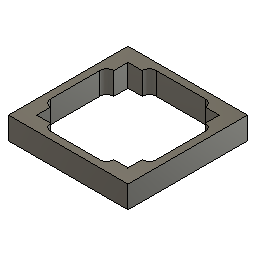
TinyNES_Foam_Bottom (Autodesk Fusion 360 design; units mm, degrees)
Autodesk Fusion 360 part; units mm, degrees
sketch "Sketch1" plane through (0, 0, 0) normal (0, 1, 0) x (1, 0, 0)
  line L0 (0, 0) -> (170, 0)
  line L1 (170, 0) -> (170, 170)
  line L2 (170, 170) -> (0, 170)
  line L3 (0, 170) -> (0, 0)
  line L4 (85, 0) -> (85, 170) construction
  line L5 (150, 150) -> (20, 150)
  line L6 (20, 150) -> (20, 20)
  line L7 (20, 20) -> (150, 20)
  line L8 (150, 20) -> (150, 150)
  line L9 (150, 150) -> (20, 20) construction
  line L10 (20, 150) -> (150, 20) construction
  line L11 (120, 160) -> (50, 160)
  line L12 (40, 150) -> (40, 20) construction
  line L13 (50, 10) -> (120, 10)
  line L14 (130, 20) -> (130, 150) construction
  line L15 (130, 160) -> (40, 10) construction
  line L16 (40, 160) -> (130, 10) construction
  line L17 (150, 130) -> (20, 130) construction
  line L18 (10, 120) -> (10, 50)
  line L19 (20, 40) -> (150, 40) construction
  line L20 (160, 50) -> (160, 120)
  line L21 (160, 130) -> (10, 40) construction
  line L22 (10, 130) -> (160, 40) construction
  arc A0 (50, 160) -> (40, 150) centre (50, 150) ccw
  arc A1 (130, 150) -> (120, 160) centre (120, 150) ccw
  arc A2 (160, 120) -> (150, 130) centre (150, 120) ccw
  arc A3 (150, 40) -> (160, 50) centre (150, 50) ccw
  arc A4 (120, 10) -> (130, 20) centre (120, 20) ccw
  arc A5 (40, 20) -> (50, 10) centre (50, 20) ccw
  arc A6 (10, 50) -> (20, 40) centre (20, 50) ccw
  arc A7 (20, 130) -> (10, 120) centre (20, 120) ccw
  point P0 (85, 85)
  point P1 (85, 85)
  point P2 (85, 85)
  dimension "d1" = 170
  dimension "d2" = 170
  dimension "d3" = 130
  dimension "d4" = 130
  dimension "d5" = 90
  dimension "d6" = 150
  dimension "d7" = 150
  dimension "d8" = 90
  dimension "d9" = 10
  dimension "d10" = 10
  dimension "d11" = 10
  dimension "d12" = 10
  dimension "d13" = 10
  dimension "d14" = 10
  dimension "d15" = 10
  dimension "d16" = 10
  constraint horizontal L0
  constraint vertical L1
  constraint horizontal L2
  constraint vertical L3
  constraint coincident L0.start L3.end
  constraint midpoint L0 L4.start
  constraint midpoint L2 L4.end
  constraint horizontal L5
  constraint perpendicular L5 L6
  constraint parallel L5 L7
  constraint parallel L6 L8
  constraint coincident L9 P2
  constraint coincident L10 P2
  constraint midpoint L4 P2
  constraint horizontal L11
  constraint perpendicular L11 L12
  constraint parallel L11 L13
  constraint parallel L12 L14
  constraint coincident L15 P2
  constraint coincident L16 P2
  constraint coincident P2 P1
  constraint horizontal L17
  constraint perpendicular L17 L18
  constraint parallel L17 L19
  constraint parallel L18 L20
  constraint coincident L21 P2
  constraint coincident L22 P2
  constraint coincident L16.start L11
  constraint coincident L16.start L12
  constraint tangent L11 A0
  constraint tangent L12 A0
  constraint coincident L15.start L11
  constraint coincident L15.start L14
  constraint tangent L11 A1
  constraint tangent L14 A1
  constraint coincident L21.start L17
  constraint coincident L21.start L20
  constraint tangent L17 A2
  constraint tangent L20 A2
  constraint coincident L22.end L20
  constraint coincident L22.end L19
  constraint tangent L20 A3
  constraint tangent L19 A3
  constraint coincident L16.end L14
  constraint coincident L16.end L13
  constraint tangent L14 A4
  constraint tangent L13 A4
  constraint coincident L15.end L13
  constraint coincident L15.end L12
  constraint tangent L13 A5
  constraint tangent L12 A5
  constraint coincident L21.end L19
  constraint coincident L21.end L18
  constraint tangent L19 A6
  constraint tangent L18 A6
  constraint coincident L22.start L18
  constraint coincident L22.start L17
  constraint tangent L18 A7
  constraint tangent L17 A7
  measures "d1" distance of L0.start L0.end
  measures "d2" distance of L0.start L2.end
  measures "d3" distance of L6.end L7.end
  measures "d4" distance of L5.end L6.end
  measures "d5" distance of L15.end L16.end
  measures "d6" distance of L16.start L15.end
  measures "d7" distance of L21.end L22.end
  measures "d8" distance of L22.start L21.end
  measures "d9" radius of A0
  measures "d10" radius of A1
  measures "d11" radius of A2
  measures "d12" radius of A3
  measures "d13" radius of A4
  measures "d14" radius of A5
  measures "d15" radius of A6
  measures "d16" radius of A7
extrude "Extrude1" add sketch "Sketch1" along normal blind 31.75
